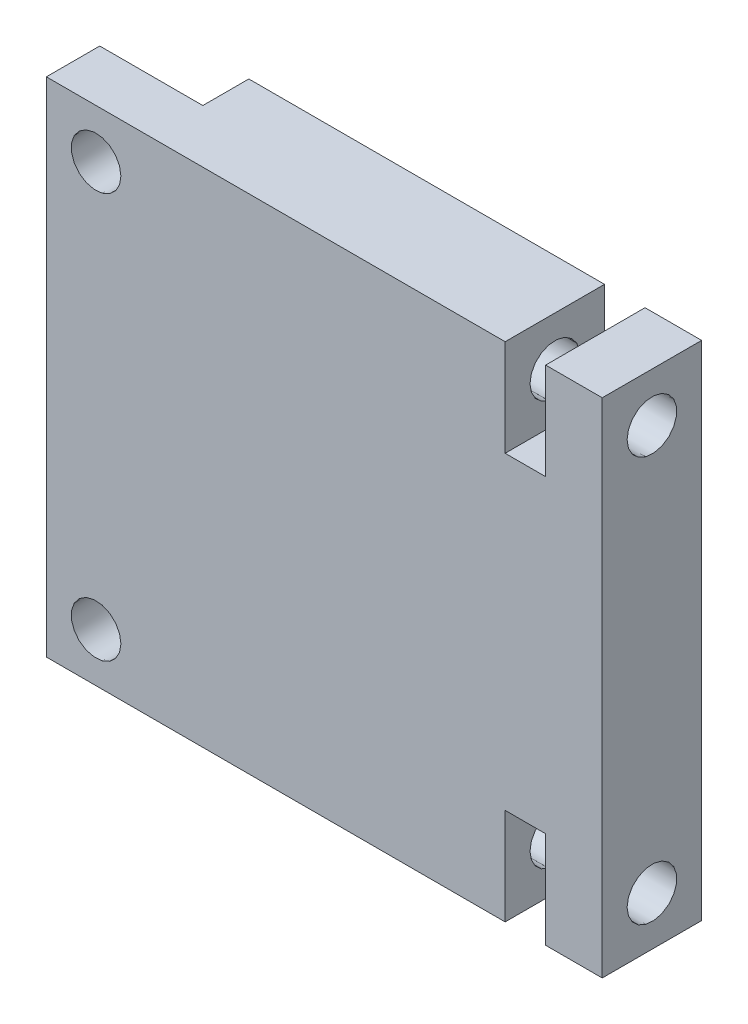
# Autodesk Inventor part: 64-106_connect
Saved by Autodesk Inventor 2024 (Build 280153000, 153)
## iProperties
Created: 2024-09-17
Part Number: 64-106_connect
Material: 일반
Document SubType Name: Modeling
Designer: Eungang
Density: 1 g/cm^3
Appearance: 기본값
Author: Eungang
Autodesk Inventor part; units mm, degrees
ref_plane "YZ Plane" through (0, 0, 0) normal (1, 0, 0) x (0, 1, 0)
ref_plane "XZ Plane" through (0, 0, 0) normal (0, 1, 0) x (-1, 0, 0)
ref_plane "XY Plane" through (0, 0, 0) normal (0, 0, 1) x (1, 0, 0)
ref_plane "작업 평면1" through (44.8, 0, -17) normal (-1, 0, 0) x (0, 0, 1)
sketch "스케치2" plane through (44.8, 0, -17) normal (-1, 0, 0) x (0, 0, 1)
  arc A0 (-19.5808, 6.2636) -> (-20.1, 4.5766) centre (-17.1, 4.5766) ccw projected
  line L0 (-20.1, -39.6766) -> (-20.1, 4.5766) projected
  arc A1 (-20.1, -39.6766) -> (-19.5808, -41.3636) centre (-17.1, -39.6766) ccw projected
  line L1 (-15.8929, -46.7869) -> (-19.5808, -41.3636) projected
  arc A2 (-15.8929, -46.7869) -> (-13.4121, -48.1) centre (-13.4121, -45.1) ccw projected
  line L2 (13.4121, -48.1) -> (-13.4121, -48.1) projected
  arc A3 (13.4121, -48.1) -> (15.8929, -46.7869) centre (13.4121, -45.1) ccw projected
  line L3 (19.5808, -41.3636) -> (15.8929, -46.7869) projected
  arc A4 (19.5808, -41.3636) -> (20.1, -39.6766) centre (17.1, -39.6766) ccw projected
  line L4 (20.1, 4.5766) -> (20.1, -39.6766) projected
  arc A5 (20.1, 4.5766) -> (19.5808, 6.2636) centre (17.1, 4.5766) ccw projected
  line L5 (15.5953, 12.1246) -> (19.5808, 6.2636) projected
  arc A6 (15.5953, 12.1246) -> (13.9414, 13) centre (13.9414, 11) ccw projected
  line L6 (7.65, 13) -> (13.9414, 13) projected
  arc A7 (9.15, 11.5) -> (7.65, 13) centre (7.65, 11.5) ccw projected
  line L7 (9.15, 11.5) -> (9.15, 10) projected
  arc A8 (9.15, 10) -> (11.5, 7.65) centre (11.5, 10) ccw projected
  line L8 (11.5, 7.65) -> (13.5, 7.65) projected
  arc A9 (14.5, 6.65) -> (13.5, 7.65) centre (13.5, 6.65) ccw projected
  line L9 (14.5, 6.65) -> (14.5, -36.15) projected
  arc A10 (13.5, -37.15) -> (14.5, -36.15) centre (13.5, -36.15) ccw projected
  line L10 (13.5, -37.15) -> (11.5, -37.15) projected
  arc A11 (11.5, -37.15) -> (9.15, -39.5) centre (11.5, -39.5) ccw projected
  line L11 (9.15, -39.5) -> (9.15, -41.5) projected
  arc A12 (8.15, -42.5) -> (9.15, -41.5) centre (8.15, -41.5) ccw projected
  line L12 (8.15, -42.5) -> (-8.15, -42.5) projected
  arc A13 (-9.15, -41.5) -> (-8.15, -42.5) centre (-8.15, -41.5) ccw projected
  line L13 (-9.15, -41.5) -> (-9.15, -39.5) projected
  arc A14 (-9.15, -39.5) -> (-11.5, -37.15) centre (-11.5, -39.5) ccw projected
  line L14 (-11.5, -37.15) -> (-13.5, -37.15) projected
  arc A15 (-14.5, -36.15) -> (-13.5, -37.15) centre (-13.5, -36.15) ccw projected
  line L15 (-14.5, -36.15) -> (-14.5, 6.65) projected
  arc A16 (-13.5, 7.65) -> (-14.5, 6.65) centre (-13.5, 6.65) ccw projected
  line L16 (-13.5, 7.65) -> (-11.5, 7.65) projected
  arc A17 (-11.5, 7.65) -> (-9.15, 10) centre (-11.5, 10) ccw projected
  line L17 (-9.15, 10) -> (-9.15, 11.5) projected
  arc A18 (-7.65, 13) -> (-9.15, 11.5) centre (-7.65, 11.5) ccw projected
  line L18 (-13.9414, 13) -> (-7.65, 13) projected
  arc A19 (-13.9414, 13) -> (-15.5953, 12.1246) centre (-13.9414, 11) ccw projected
  line L19 (-19.5808, 6.2636) -> (-15.5953, 12.1246) projected
  circle A20 centre (17.3, 4) radius 1.35 projected
  circle A21 centre (17.3, -18) radius 1.35 projected
  circle A22 centre (11, -45.3) radius 1.35 projected
  circle A23 centre (-17.3, 4) radius 1.35 projected
  circle A24 centre (-17.3, -18) radius 1.35 projected
  circle A25 centre (-11, -45.3) radius 1.35 projected
  circle A26 centre (17.3, -40) radius 1.35 projected
  circle A27 centre (-17.3, -40) radius 1.35 projected
  line L20 (17.3, -19.35) -> (17.3, 5.35)
  line L21 (20.1, 4.5766) -> (20.1, 6.65)
  line L22 (20.1, 6.65) -> (14.5, 6.65)
  line L23 (17.3, -7) -> (20.1, -7)
  arc A28 (19.5808, -20.2636) -> (20.1, -18.5766) centre (17.1, -18.5766) ccw
  line L24 (20.1, -18.5766) -> (20.1, -20.65)
  line L25 (20.1, -20.65) -> (14.5, -20.65)
  line L26 (20.1, -20.65) -> (14.5, -20.65)
  line L27 (14.5, -20.65) -> (14.5, 6.65)
  line L28 (14.5, 6.65) -> (20.1, 6.65)
  line L29 (20.1, 6.65) -> (20.1, -20.65)
  line L30 (14.6, -36.15) -> (14.6, 6.65)
  arc A29 (14.6, 6.65) -> (13.5, 7.75) centre (13.5, 6.65) ccw
  line L31 (13.5, 7.75) -> (11.5, 7.75)
  arc A30 (9.25, 10) -> (11.5, 7.75) centre (11.5, 10) ccw
  line L32 (9.25, 10) -> (9.25, 11.5)
  arc A31 (9.25, 11.5) -> (8.4246, 12.9) centre (7.65, 11.5) ccw
  line L33 (8.4246, 12.9) -> (13.9414, 12.9)
  arc A32 (15.5126, 12.0684) -> (13.9414, 12.9) centre (13.9414, 11) ccw
  line L34 (15.5126, 12.0684) -> (19.4981, 6.2073)
  arc A33 (20, 4.5766) -> (19.4981, 6.2073) centre (17.1, 4.5766) ccw
  line L35 (20, 4.5766) -> (20, -39.6766)
  arc A34 (19.4981, -41.3073) -> (20, -39.6766) centre (17.1, -39.6766) ccw
  line L36 (19.4981, -41.3073) -> (15.8102, -46.7307)
  arc A35 (13.4121, -48) -> (15.8102, -46.7307) centre (13.4121, -45.1) ccw
  line L37 (13.4121, -48) -> (-13.4121, -48)
  arc A36 (-15.8102, -46.7307) -> (-13.4121, -48) centre (-13.4121, -45.1) ccw
  line L38 (-15.8102, -46.7307) -> (-19.4981, -41.3073)
  arc A37 (-20, -39.6766) -> (-19.4981, -41.3073) centre (-17.1, -39.6766) ccw
  line L39 (-20, -39.6766) -> (-20, 4.5766)
  arc A38 (-19.4981, 6.2073) -> (-20, 4.5766) centre (-17.1, 4.5766) ccw
  line L40 (-19.4981, 6.2073) -> (-15.5126, 12.0684)
  arc A39 (-13.9414, 12.9) -> (-15.5126, 12.0684) centre (-13.9414, 11) ccw
  line L41 (-13.9414, 12.9) -> (-8.4246, 12.9)
  arc A40 (-8.4246, 12.9) -> (-9.25, 11.5) centre (-7.65, 11.5) ccw
  line L42 (-9.25, 11.5) -> (-9.25, 10)
  arc A41 (-11.5, 7.75) -> (-9.25, 10) centre (-11.5, 10) ccw
  line L43 (-11.5, 7.75) -> (-13.5, 7.75)
  arc A42 (-13.5, 7.75) -> (-14.6, 6.65) centre (-13.5, 6.65) ccw
  line L44 (-14.6, 6.65) -> (-14.6, -36.15)
  arc A43 (-14.6, -36.15) -> (-13.5, -37.25) centre (-13.5, -36.15) ccw
  line L45 (-13.5, -37.25) -> (-11.5, -37.25)
  arc A44 (-9.25, -39.5) -> (-11.5, -37.25) centre (-11.5, -39.5) ccw
  line L46 (-9.25, -39.5) -> (-9.25, -41.5)
  arc A45 (-9.25, -41.5) -> (-8.15, -42.6) centre (-8.15, -41.5) ccw
  line L47 (-8.15, -42.6) -> (8.15, -42.6)
  arc A46 (8.15, -42.6) -> (9.25, -41.5) centre (8.15, -41.5) ccw
  line L48 (9.25, -41.5) -> (9.25, -39.5)
  arc A47 (11.5, -37.25) -> (9.25, -39.5) centre (11.5, -39.5) ccw
  line L49 (11.5, -37.25) -> (13.5, -37.25)
  arc A48 (13.5, -37.25) -> (14.6, -36.15) centre (13.5, -36.15) ccw
  line L50 (20, 4.5766) -> (20, 6.65)
  line L51 (17, 8.5) -> (17, -44.6) projected
  line L52 (17, 8.5) -> (17, -44.6) projected
  point P0 (17, 0)
  point P1 (17.3, -18)
  point P2 (14.6, -20.65)
  point P3 (20, -20.65)
  dimension "d3" = 0.1
  constraints: 62 end point, 42 point on circle, 21 centre point, 6 symmetric about line, 4 perpendicular, 3 parallel, 2 point on line, 2 vertical alignment, 1 horizontal, 1 midpoint, 1 vertical, 42 other
  measures "d3" distance between parallel lines of L9 L30
extrude "돌출2" add sketch "스케치2" along normal blind 24.6 contours L25 L51 A21 L20 L23 L35 | L25 L30 L22 L51 A20 A21 | L23 L20 A20 L51 L22 L34 A33 L35 | L50 A33 L34 L22 L5 A5 | A5 L5 L22 L50 | L20 A21 L51 A20
sketch "스케치3" plane through (20.2, 0, -17) normal (-1, 0, 0) x (0, 0, 1)
  line L0 (17, 8.5) -> (17, -44.6) projected
  line L1 (14.6, -20.65) -> (20, -20.65) projected
  line L2 (20, -20.65) -> (20, 6.65) projected
  line L3 (17, -20.65) -> (20, -20.65)
  line L4 (20, -20.65) -> (20, 6.65)
  line L5 (20, 6.65) -> (17, 6.65)
  line L6 (17, 6.65) -> (17, -20.65)
  line L7 (17.1, 8.5) -> (17.1, -44.6)
  point P0 (17, 0)
  point P1 (17.1, 6.65)
  point P2 (17.1, -20.65)
  dimension "d6" = 0.1
  constraints: 10 end point, 3 parallel, 2 point on line, 1 horizontal, 1 perpendicular
  measures "d6" distance between parallel lines of L0 L7
extrude "돌출3" add sketch "스케치3" along normal blind 5.6 contours L5 L2 L1 L7
sketch "스케치4" plane through (44.8, -20.65, 3) normal (0, 0, 1) x (1, 0, 0)
  line L0 (-31.3, -19.1) -> (-33.3, -19.1) projected
  arc A0 (-33.3, -19.1) -> (-35.55, -21.35) centre (-33.3, -21.35) ccw projected
  line L1 (-35.55, -21.35) -> (-35.55, -23.35) projected
  arc A1 (-36.55, -24.35) -> (-35.55, -23.35) centre (-36.55, -23.35) ccw projected
  line L2 (-36.55, -24.35) -> (-53.05, -24.35) projected
  arc A2 (-54.05, -23.35) -> (-53.05, -24.35) centre (-53.05, -23.35) ccw projected
  line L3 (-54.05, -23.35) -> (-54.05, -21.35) projected
  arc A3 (-54.05, -21.35) -> (-56.3, -19.1) centre (-56.3, -21.35) ccw projected
  line L4 (-56.3, -19.1) -> (-58.3, -19.1) projected
  arc A4 (-59.3, -18.1) -> (-58.3, -19.1) centre (-58.3, -18.1) ccw projected
  line L5 (-59.3, -18.1) -> (-59.3, 28.9) projected
  arc A5 (-58.3, 29.9) -> (-59.3, 28.9) centre (-58.3, 28.9) ccw projected
  line L6 (-58.3, 29.9) -> (-56.3, 29.9) projected
  arc A6 (-56.3, 29.9) -> (-54.05, 32.15) centre (-56.3, 32.15) ccw projected
  line L7 (-54.05, 32.15) -> (-54.05, 35.15) projected
  line L8 (-59.8, 35.15) -> (-54.05, 35.15) projected
  line L9 (-64.9, 29.15) -> (-59.8, 35.15) projected
  line L10 (-64.9, -23.95) -> (-64.9, 29.15) projected
  line L11 (-59.8, -29.95) -> (-64.9, -23.95) projected
  line L12 (-29.8, -29.95) -> (-59.8, -29.95) projected
  line L13 (-24.7, -23.95) -> (-29.8, -29.95) projected
  line L14 (-24.7, 29.15) -> (-24.7, -23.95) projected
  line L15 (-29.8, 35.15) -> (-24.7, 29.15) projected
  line L16 (-35.55, 35.15) -> (-29.8, 35.15) projected
  line L17 (-35.55, 35.15) -> (-35.55, 32.15) projected
  arc A7 (-35.55, 32.15) -> (-33.3, 29.9) centre (-33.3, 32.15) ccw projected
  line L18 (-33.3, 29.9) -> (-31.3, 29.9) projected
  arc A8 (-30.3, 28.9) -> (-31.3, 29.9) centre (-31.3, 28.9) ccw projected
  line L19 (-30.3, 28.9) -> (-30.3, -18.1) projected
  arc A9 (-31.3, -19.1) -> (-30.3, -18.1) centre (-31.3, -18.1) ccw projected
  circle A10 centre (-27.5, 24.65) radius 1.35 projected
  circle A11 centre (-27.5, 2.65) radius 1.35 projected
  circle A12 centre (-33.8, -27.15) radius 1.35 projected
  circle A13 centre (-62.1, 24.65) radius 1.35 projected
  circle A14 centre (-62.1, 2.65) radius 1.35 projected
  circle A15 centre (-55.8, -27.15) radius 1.35 projected
  circle A16 centre (-27.5, -19.35) radius 1.35 projected
  circle A17 centre (-62.1, -19.35) radius 1.35 projected
  point P0 (-44.8, 20.65)
extrude "돌출4" cut sketch "스케치4" against normal up to next contours A10 | A11
sketch "스케치5" plane through (44.8, -20.65, 3) normal (0, 0, 1) x (1, 0, 0)
  line L0 (-5.275, 23.4) -> (2.4, 23.4)
  line L1 (-5.275, 25.9) -> (2.4, 25.9)
  line L2 (-5.275, 23.4) -> (-5.275, 25.9)
  line L3 (-5.275, 24.65) -> (2.4, 24.65)
  line L4 (-5.275, 24.65) -> (-3.075, 24.65)
  line L5 (-3.075, 24.65) -> (-3.075, 22.05)
  line L6 (-3.075, 22.05) -> (-5.275, 22.05)
  line L7 (-5.275, 22.05) -> (-5.275, 24.65)
  line L8 (-3.075, 24.65) -> (-3.075, 27.25)
  line L9 (-3.075, 27.25) -> (-5.275, 27.25)
  line L10 (-5.275, 27.25) -> (-5.275, 24.65)
  line L11 (0, 27.3) -> (-30.2, 27.3) projected
  line L12 (-3.075, 27.25) -> (-5.275, 27.25)
  line L13 (-5.275, 27.25) -> (-5.275, 27.3)
  line L14 (-5.275, 27.3) -> (-3.075, 27.3)
  line L15 (-3.075, 27.3) -> (-3.075, 27.25)
  circle A0 centre (-27.5, 24.65) radius 1.35 projected
  circle A1 centre (-27.5, 2.65) radius 1.35 projected
  line L16 (0, 0) -> (0, 27.3) projected
  line L17 (0, 27.3) -> (-30.2, 27.3) projected
  line L18 (-30.2, 0) -> (-30.2, 27.3) projected
  line L19 (0, 0) -> (-30.2, 0) projected
  line L20 (0, 13.65) -> (-30.2, 13.65)
  line L21 (-5.275, 3.9) -> (-5.275, 1.4)
  line L22 (-5.275, 2.65) -> (-3.075, 2.65)
  line L23 (-3.075, 2.65) -> (-3.075, 5.25)
  line L24 (-3.075, 5.25) -> (-5.275, 5.25)
  line L25 (-5.275, 5.25) -> (-5.275, 2.65)
  line L26 (-3.075, 2.65) -> (-3.075, 0.05)
  line L27 (-3.075, 0.05) -> (-5.275, 0.05)
  line L28 (-5.275, 0.05) -> (-5.275, 2.65)
  line L29 (-3.075, 0.05) -> (-5.275, 0.05)
  line L30 (-5.275, 0.05) -> (-5.275, 0)
  line L31 (-5.275, 0) -> (-3.075, 0)
  line L32 (-3.075, 0) -> (-3.075, 0.05)
  point P0 (-44.8, 20.65)
  point P1 (-3.075, 27.3)
  point P2 (-5.275, 27.25)
  point P3 (-5.275, 25.9)
  point P4 (-5.275, 23.4)
  point P5 (-5.275, 0.05)
  point P6 (-5.275, 0)
  point P7 (-3.075, 0)
  point P8 (-5.275, 3.9)
  point P9 (-5.275, 1.4)
  dimension "d11" = 2.2
  dimension "d12" = 2.6
  constraints: 56 end point, 13 symmetric about line, 5 horizontal, 4 parallel, 3 midpoint, 2 perpendicular, 1 point on line, 4 other
  measures "d11" distance of L5.end L6.end
  measures "d12" distance between parallel lines of L3 L6
extrude "돌출5" cut sketch "스케치5" against normal blind 10 contours L2 L3 L5 L0 | L0 L5 L6 L7 | L2 L1 L8 L3 | L10 L9 L8 L1 | L13 L11 L15 L9 | L19 L30 L27 L32 | L27 L28 L21 L22 L26 | L22 L21 L25 L24 L23
